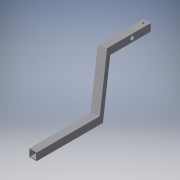
# Autodesk Inventor part: Arm 2
Saved by Autodesk Inventor 2017 (Build 210142000, 142)
## iProperties
Created: 2019-02-04
Part Number: Arm 2
Material: Generic
Document SubType Name: Modeling
Designer: S346553810
Density: 1 g/cm^3
Appearance: Default
Author: S346553810
Autodesk Inventor part; units mm, degrees
ref_plane "YZ Plane" through (0, 0, 0) normal (1, 0, 0) x (0, 1, 0)
ref_plane "XZ Plane" through (0, 0, 0) normal (0, 1, 0) x (-1, 0, 0)
ref_plane "XY Plane" through (0, 0, 0) normal (0, 0, 1) x (1, 0, 0)
sketch "Sketch1" plane through (0, 0, 0) normal (0, 0, 1) x (1, 0, 0)
  line L0 (0, 0) -> (-25.4, 0)
  line L1 (-25.4, 0) -> (-25.4, 25.4)
  line L2 (-25.4, 25.4) -> (0, 25.4)
  line L3 (0, 25.4) -> (0, 0)
  line L4 (-2.54, 22.86) -> (-22.86, 22.86)
  line L5 (-22.86, 22.86) -> (-22.86, 2.54)
  line L6 (-22.86, 2.54) -> (-2.54, 2.54)
  line L7 (-2.54, 2.54) -> (-2.54, 22.86)
  dimension "d0" = 25.4
  dimension "d1" = 25.4
  dimension "d2" = 2.54
  constraints: 16 end point, 4 parallel, 2 perpendicular, 1 horizontal, 3 other
  measures "d0" distance of L1.end L2.end
  measures "d1" distance of L0.end L1.end
  measures "d2" distance between parallel lines of L2 L4
sketch "Sketch2" plane through (0, 0, 0) normal (1, 0, 0) x (0, 1, 0)
  line L0 (0, 0) -> (0, -304.8)
  line L1 (0, -304.8) -> (114.3, -406.4)
  line L2 (0, -304.8) -> (152.9283, -304.8) construction
  line L3 (114.3, -406.4) -> (114.3, -546.1)
  dimension "d3" = 304.8
  dimension "d5" = 139.7
  dimension "d6" = 114.3
  dimension "d7" = 101.6
  constraints: 8 end point, 2 vertical, 1 equal length, 1 horizontal
  measures "d3" distance of L0.start L0.end
  measures "d5" distance of L1.end L3.end
  measures "d6" distance between parallel lines of L0 L3
  measures "d7" vertical distance of L0.end L1.end
sketch "Sketch3" plane through (0, 0, 0) normal (0, 1, 0) x (-1, 0, 0)
  line L0 (0, -406.4) -> (0, -546.1) projected
  line L1 (0, 0) -> (0, -304.8) projected
  line L2 (0, -304.8) -> (76.2, -406.4)
  line L3 (76.2, -406.4) -> (76.2, -546.1)
  dimension "d8" = 76.2
  constraints: 4 end point, 2 horizontal alignment, 1 vertical
  measures "d8" distance between parallel lines of L0 L3
sketch3d "3D Sketch3"
  line L0 (0, 0, 0) -> (0, 0, -304.8)
  line L1 (0, 0, -304.8) -> (-76.2, 114.3, -406.4)
  line L2 (-76.2, 114.3, -406.4) -> (-76.2, 114.3, -546.1)
sweep "Sweep1" add profiles "Sketch1" path "3D Sketch3"
sketch "Sketch6" plane through (-76.2, 114.3, -546.1) normal (1, 0, 0) x (0, 0, -1)
  circle A0 centre (-63.5, 12.7) radius 6.35
  line L0 (0, 25.4) -> (0, 0) projected
  point P0 (-546.1, -114.3)
  dimension "d19" = 12.7
  dimension "d20" = 63.5
  constraints: 1 centre point
  measures "d19" diameter of A0
  measures "d20" distance from line of L0 A0.centre
extrude "Extrusion3" cut sketch "Sketch6" against normal through all
sketch "Sketch7" plane through (-101.6, 139.7, -546.1) normal (0, 1, 0) x (1, 0, 0)
  circle A0 centre (12.7, -12.7) radius 3.175
  line L0 (0, -157.4592) -> (0, 0) projected
  line L1 (0, 0) -> (25.4, 0) projected
  point P0 (101.6, -546.1)
  dimension "d23" = 6.35
  dimension "d24" = 12.7
  dimension "d25" = 12.7
  constraints: 1 centre point
  measures "d23" diameter of A0
  measures "d24" distance from line of L0 A0.centre
  measures "d25" distance from line of L1 A0.centre
extrude "Extrusion4" cut sketch "Sketch7" against normal through all
body "Solid1"
